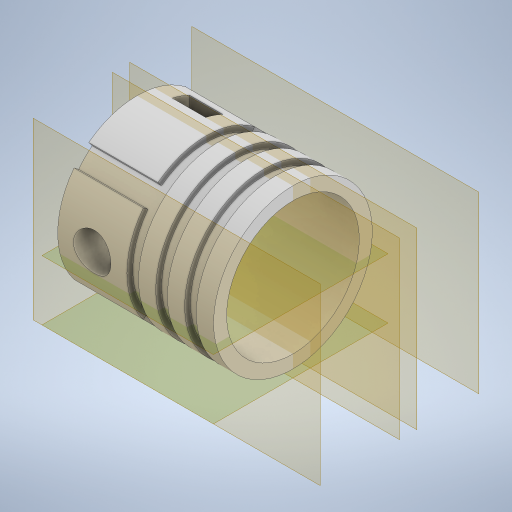
# Autodesk Inventor part: kolo_tetsowe
Saved by Autodesk Inventor 2023.5 (Build 275446000, 446)
## iProperties
Created: 2025-01-11
Part Number: kolo_tetsowe
Material: Ogólny
Document SubType Name: Modeling
Designer: kamil
Density: 1 g/cm^3
Appearance: Domyślna
Author: kamil
Autodesk Inventor part; units mm, degrees
ref_plane "YZ Plane" through (0, 0, 0) normal (1, 0, 0) x (0, 1, 0)
ref_plane "XZ Plane" through (0, 0, 0) normal (0, 1, 0) x (-1, 0, 0)
sketch "Szkic1" plane through (0, 0, 0) normal (1, 0, 0) x (0, 1, 0)
  circle A0 centre (0, 0) radius 16
  dimension "d0" = 32
  constraints: 1 centre point, 1 coincident
  measures "d0" diameter of A0
extrude "Wyciągnięcie proste1" add sketch "Szkic1" along normal blind 28
sketch "Szkic2" plane through (0, 0, 0) normal (-1, 0, 0) x (0, 0, 1)
  circle A0 centre (0, 0) radius 11.5
  dimension "d3" = 23
  constraints: 1 centre point, 1 coincident
  measures "d3" diameter of A0
extrude "Wyciągnięcie proste2" cut sketch "Szkic2" against normal blind 30.8
sketch "Szkic3" plane through (0, 0, 0) normal (-1, 0, 0) x (0, 0, 1)
  circle A0 centre (0, 0) radius 16 projected
extrude "Wyciągnięcie proste3" add sketch "Szkic3" against normal blind 2
sketch "Szkic4" plane through (0, 0, 0) normal (-1, 0, 0) x (0, 0, 1)
  circle A0 centre (0, 0) radius 1.8
  dimension "d8" = 3.6
  constraints: 1 centre point, 1 coincident
  measures "d8" diameter of A0
extrude "Wyciągnięcie proste4" cut sketch "Szkic4" against normal blind 28
sketch "Szkic5" plane through (2, 0, 0) normal (1, 0, 0) x (0, 0, -1)
  circle A0 centre (0, 0) radius 1.8 projected
  circle A1 centre (0, 0) radius 11.5 projected
extrude "Wyciągnięcie proste5" add sketch "Szkic5" along normal blind 9
sketch "Szkic6" plane through (28, 0, 0) normal (1, 0, 0) x (0, 0, -1)
  circle A0 centre (0, 0) radius 11.5 projected
  circle A1 centre (0, 0) radius 16 projected
  line L0 (-11.5, 0) -> (-16, 0)
  circle A2 centre (0, 0) radius 13.75
  point P0 (-13.75, 0)
  constraints: 4 horizontal alignment, 2 end point, 1 coincident, 1 horizontal, 1 midpoint, 4 other
extrude "Wyciągnięcie proste6" cut sketch "Szkic6" against normal through all contours A1
sketch "Szkic7" plane through (28, 0, 0) normal (1, 0, 0) x (0, 0, -1)
  circle A0 centre (0, 0) radius 13.75 projected
  circle A1 centre (0, 0) radius 11.5 projected
extrude "Wyciągnięcie proste7" add sketch "Szkic7" along normal blind 1
ref_plane "Płaszczyzna konstrukcyjna1" through (28, 0, 0) normal (0, 0, 1) x (1, 0, 0)
sketch "Szkic8" plane through (28, 0, 0) normal (0, 0, 1) x (1, 0, 0)
  line L0 (1, -13.75) -> (1, 13.75) projected
  line L1 (-28, 13.75) -> (-28, -13.75) projected
  line L2 (1, 11.5) -> (1, -11.5) projected
  line L3 (-17, 11.5) -> (-17, -11.5) projected
  line L4 (-19, 7.6749) -> (-19, -7.6749)
  line L5 (-28, 13.75) -> (1, 13.75) projected
  line L6 (-28, 13.75) -> (-19, 13.75)
  line L7 (-19, 13.75) -> (-19, 11.75)
  line L8 (-19, 11.75) -> (-28, 11.75)
  line L9 (-28, 11.75) -> (-28, 13.75)
  line L10 (-26, 11.75) -> (-26, 13.75)
  line L11 (-23.5, 13.75) -> (-23.5, 11.75)
  line L12 (-21.5, 13.75) -> (-21.5, 11.75)
  line L13 (-28, 0) -> (-19, 0)
  point P0 (-17, 0)
  point P1 (-19, 13.75)
  dimension "d17" = 2
  dimension "d18" = 2
  dimension "d19" = 2
  dimension "d20" = 2.5
  dimension "d21" = 2.5
  constraints: 18 end point, 5 point on line, 4 midpoint, 4 perpendicular, 3 parallel, 1 horizontal, 1 horizontal alignment
  measures "d17" distance between parallel lines of L3 L4
  measures "d18" distance of L6.end L7.end
  measures "d19" distance between parallel lines of L1 L10
  measures "d20" distance from line of L4.start L12
  measures "d21" distance between parallel lines of L10 L11
revolve "Obrót1" [suppressed]
sketch "Szkic9" plane through (11, 0, 0) normal (1, 0, 0) x (0, 0, -1)
  circle A0 centre (0, 0) radius 11.5 projected
  circle A1 centre (0, 0) radius 1.8 projected
extrude "Wyciągnięcie proste8" add sketch "Szkic9" along normal blind 0.5
sketch "Szkic10" plane through (28, 0, 0) normal (0, 0, 1) x (1, 0, 0)
  line L0 (-23.15, -1) -> (-23.15, 1) projected
  line L1 (-16.9, 1) -> (-16.9, -1) projected
  line L2 (-23.15, 0) -> (-16.9, 0)
  circle A0 centre (-20.025, 0) radius 1.4
  point P0 (-28, 0)
  dimension "d25" = 2.8
  constraints: 3 midpoint, 2 end point, 1 centre point
  measures "d25" diameter of A0
extrude "Wyciągnięcie proste9" cut sketch "Szkic10" along normal mid plane 30
ref_plane "Płaszczyzna konstrukcyjna2" through (28, 0, -13.75) normal (0, 0, 1) x (1, 0, 0)
sketch "Szkic11" plane through (28, 0, -13.75) normal (0, 0, 1) x (1, 0, 0)
  circle A0 centre (-20.025, 0) radius 1.4
  point P0 (-28, 0)
  constraints: 2 coincident, 1 centre point, 2 other
hole "Otwór1" at (7.975, 0, -13.75) direction (0, 0, 1) diameter 3.2 end through all counterbore diameter 6.5 counterbore depth 6
ref_plane "Płaszczyzna konstrukcyjna3" through (28, 0, -3) normal (0, 0, 1) x (1, 0, 0)
sketch "Szkic12" plane through (28, 0, -3) normal (0, 0, 1) x (1, 0, 0)
  circle A0 centre (-20.025, 0) radius 1.6 projected
  circle A1 centre (-20.025, 0) radius 2.9
  line L0 (-22.925, 1.6743) -> (-20.025, 3.3486)
  line L1 (-20.025, 3.3486) -> (-17.125, 1.6743)
  line L2 (-17.125, 1.6743) -> (-17.125, -1.6743)
  line L3 (-17.125, -1.6743) -> (-20.025, -3.3486)
  line L4 (-20.025, -3.3486) -> (-22.925, -1.6743)
  line L5 (-22.925, -1.6743) -> (-22.925, 1.6743)
  line L6 (-22.925, 17.3819) -> (-17.125, 17.3819)
  line L7 (-17.125, 17.3819) -> (-17.125, 1.6743)
  line L8 (-17.125, 1.6743) -> (-22.925, 1.6743)
  line L9 (-22.925, 1.6743) -> (-22.925, 17.3819)
  point P0 (-28, 0)
  point P1 (-22.925, 0)
  dimension "d36" = 5.8
  constraints: 20 end point, 2 coincident, 2 parallel, 1 horizontal, 1 horizontal alignment, 1 midpoint, 1 perpendicular, 15 other
extrude "Wyciągnięcie proste10" cut sketch "Szkic12" against normal blind 3 contours A0 | A1 L8 | L2 L3 A1 | A1 L8 L2 | L8 A1 | A1 L1 L8 | L3 L4 A1 | L1 L0 L9 L6 L7 | A1 L0 L1 | L8 L0 A1 | A1 L5 L8 | L4 L5 A1
sketch "Szkic13" plane through (28, 0, 0) normal (0, 0, 1) x (1, 0, 0)
  line L0 (-28, 13.75) -> (1, 13.75) projected
  line L1 (-16.5, 11.5) -> (-16.5, -11.5) projected
  line L2 (1, 11.5) -> (1, -11.5) projected
  line L3 (1, 0) -> (-16.5, 0)
  line L4 (-16.5, 1.8) -> (-16.5, -1.8) projected
  line L5 (-2, 13.75) -> (-4, 13.75)
  line L6 (-4, 13.75) -> (-4, 12.75)
  line L7 (-4, 12.75) -> (-2, 12.75)
  line L8 (-2, 12.75) -> (-2, 13.75)
  line L9 (-7, 13.75) -> (-9, 13.75)
  line L10 (-9, 13.75) -> (-9, 12.75)
  line L11 (-9, 12.75) -> (-7, 12.75)
  line L12 (-7, 12.75) -> (-7, 13.75)
  line L13 (-12, 13.75) -> (-14, 13.75)
  line L14 (-14, 13.75) -> (-14, 12.75)
  line L15 (-14, 12.75) -> (-12, 12.75)
  line L16 (-12, 12.75) -> (-12, 13.75)
  point P0 (-28, 0)
  point P1 (-2, 13.25)
  point P2 (-7, 13.25)
  point P3 (-12, 13.25)
  point P4 (-9, 13.25)
  point P5 (-14, 13.75)
  point P6 (-9, 13.75)
  point P7 (-4, 13.75)
  dimension "d39" = 2
  dimension "d40" = 1
  dimension "d41" = 2
  dimension "d42" = 1
  dimension "d43" = 2
  dimension "d44" = 1
  dimension "d45" = 3
  dimension "d46" = 3
  dimension "d47" = 3
  constraints: 26 end point, 6 midpoint, 6 parallel, 3 horizontal, 3 perpendicular, 3 point on line
  measures "d39" distance of L7.end L6.end
  measures "d40" distance of L6.end L5.end
  measures "d41" distance of L11.end L10.end
  measures "d42" distance of L10.end L9.end
  measures "d43" distance of L15.end L14.end
  measures "d44" distance of L14.end L13.end
  measures "d45" horizontal distance of point (-2, 13.25) L0.end
  measures "d46" distance from line of point (-7, 13.25) L6
  measures "d47" distance of point (-12, 13.25) point (-9, 13.25)
revolve "Obrót2" cut sketch "Szkic13" angle 360 about axis through (29, 0, 0) along (-1, 0, 0)
fillet "Zaokrąglenie1" radius 1 1 edges at (11.5, 0, -11.5)
ref_plane "Płaszczyzna konstrukcyjna4" through (28, 0, 13.75) normal (0, 0, 1) x (1, 0, 0)
sketch "Szkic14" plane through (28, 0, 13.75) normal (0, 0, 1) x (1, 0, 0)
  circle A0 centre (-20.025, 0) radius 1.4
  point P0 (-28, 0)
  dimension "d50" = 2.8
  constraints: 2 coincident, 1 centre point, 1 other
  measures "d50" diameter of A0
hole "Otwór2" at (7.975, 0, 13.75) direction (0, 0, -1) diameter 2.8 depth 14 tip angle 118 counterbore diameter 6.5 counterbore depth 5
sketch "Szkic15" plane through (0, 0, 0) normal (-1, 0, 0) x (0, 0, 1)
  circle A0 centre (0, 0) radius 13.75 projected
  circle A1 centre (0, 0) radius 1.8 projected
extrude "Wyciągnięcie proste11" cut sketch "Szkic15" against normal blind 2
ref_plane "Płaszczyzna konstrukcyjna8" through (28, -13.75, 0) normal (0, -1, 0) x (0, 0, -1)
ref_plane "Płaszczyzna konstrukcyjna7" through (7.975, -3.3486, -3) normal (0, -1, 0) x (0, 0, -1)
sketch "Szkic16" plane through (28, -13.75, 0) normal (0, -1, 0) x (0, 0, -1)
  line L0 (-8.75, -18.625) -> (-8.75, -21.425) projected
  line L1 (-1.8, -26) -> (1.8, -26) projected
  line L2 (-1.8, -16.5) -> (1.8, -16.5) projected
  line L3 (-1.8, -16.5) -> (1.8, -16.5) projected
  line L4 (-1.8, -26) -> (1.8, -26) projected
  line L5 (0, -26) -> (0, -16.5)
  line L6 (-8.75, -16.775) -> (-8.75, -23.275) projected
  line L7 (-8.75, -20.025) -> (0, -20.025)
  point P0 (0, -28)
  point P1 (-1.1314, -20.025)
  point P2 (0.8246, -20.025)
  constraints: 4 end point, 3 midpoint, 1 coincident, 1 perpendicular, 1 point on line
hole "Otwór3" at (7.975, -13.75, 0) direction (0, 1, 0) diameter 2.8 depth 14 tip angle 118 counterbore diameter 6.5 counterbore depth 5
sketch "Szkic17" plane through (2, 0, 0) normal (-1, 0, 0) x (0, 0, 1)
  circle A0 centre (0, 0) radius 13.75 projected
  circle A1 centre (0, 0) radius 12.75
  line L0 (0, 0) -> (10.9086, 8.3705)
  line L1 (0, 0) -> (8.3705, 10.9086)
  line L2 (0, 0) -> (12.75, 0)
  point P0 (7.7617, 10.1153)
  point P1 (10.1153, 7.7617)
  dimension "d68" = 1
  dimension "d69" = 15
  dimension "d70" = 37.5
  constraints: 6 end point, 2 point on circle, 1 horizontal, 3 other
  measures "d69" angle of L1 L0
  measures "d70" angle of L0 L2
extrude "Wyciągnięcie proste12" cut sketch "Szkic17" against normal up to surface (14 mm away) contours L0 A1 L1 A0 picked at (10.3871, 8.4739)
pattern_circular "Szyk kołowy1" count 4 over 360 about axis through (28, 0, 0) along (-1, 0, 0) of "Wyciągnięcie proste12"
sketch "Szkic18" plane through (2, 0, 0) normal (-1, 0, 0) x (0, 0, 1)
  circle A0 centre (0, 0) radius 1 projected
  circle A1 centre (0, 0) radius 1.8 projected
  circle A2 centre (0, 0) radius 1.2494
  constraints: 1 centre point
ref_plane "Płaszczyzna konstrukcyjna9" through (4.85, -1.8, -1.8) normal (-1, 0, 0) x (0, 0, 1)
extrude "Wyciągnięcie proste13" add sketch "Szkic18" against normal up to surface (2.85 mm away) contours A1
sketch "Szkic19" plane through (11.5, 0, 0) normal (1, 0, 0) x (0, 0, -1)
  circle A0 centre (0, 0) radius 1.8 projected
  circle A1 centre (0, 0) radius 1.9
  dimension "d78" = 0.1
  constraints: 1 centre point
  measures "d78" radial gap between concentric circles of A0 A1
extrude "Wyciągnięcie proste14" cut sketch "Szkic19" against normal up to surface (6.65 mm away) contours A0 | A1
chamfer "Faza1" distance 0.5 angle 45 1 edges at (11.5, 0, 1.9)
chamfer "Faza2" distance 0.5 angle 45 2 edges at (7.975, -1.6, -7.75) (7.975, -8.75, 1.4)
sketch "Szkic20" plane through (11.5, 0, 0) normal (1, 0, 0) x (0, 0, -1)
  circle A0 centre (0, 0) radius 2.4 projected
extrude "Wyciągnięcie proste15" add sketch "Szkic20" against normal up to surface (9.5 mm away)
sketch "Szkic21" plane through (2, 0, 0) normal (-1, 0, 0) x (0, 0, 1)
  circle A0 centre (0, 0) radius 1.5
  line L0 (-1, 1.118) -> (-1, -1.118)
  dimension "d89" = 3
  dimension "d90" = 1
  constraints: 2 end point, 2 point on circle, 1 centre point, 1 coincident, 1 vertical
  measures "d89" diameter of A0
  measures "d90" distance from line of L0 point (0, 0)
extrude "Wyciągnięcie proste16" cut sketch "Szkic21" against normal through all contours A0 L0 picked at (-0.1667, 0)
sketch "Szkic22" plane through (7.975, 0, -7.75) normal (0, 0, -1) x (-1, 0, 0)
  circle A0 centre (0, 0) radius 1.6 projected
  point P0 (7.975, 0)
extrude "Wyciągnięcie proste17" cut sketch "Szkic22" against normal through all
sketch "Szkic23" plane through (7.975, -8.75, 0) normal (0, -1, 0) x (1, 0, 0)
  circle A0 centre (0, 0) radius 1.4 projected
  point P0 (-7.975, 0)
extrude "Wyciągnięcie proste18" cut sketch "Szkic23" against normal blind 8
sketch "Szkic24" plane through (2, 0, 0) normal (-1, 0, 0) x (0, 0, 1)
  arc A0 (-1, -1.118) -> (-1, 1.118) centre (0, 0) ccw projected
  line L0 (-1, -1.118) -> (-1, 1.118) projected
  arc A1 (-1.2, -1.2042) -> (-1.2, 1.2042) centre (0, 0) ccw
  line L1 (-1.2, -1.2042) -> (-1.2, 1.2042)
  dimension "d97" = 0.2
  constraints: 2 end point, 2 point on circle, 1 centre point, 1 other
  measures "d97" radial gap between concentric circles of A0 A1
extrude "Wyciągnięcie proste19" cut sketch "Szkic24" against normal through all contours L0 A0 | L1 A1
sketch "Szkic25" plane through (11.5, 0, 0) normal (1, 0, 0) x (0, 0, -1)
  line L0 (7.9941, 15.6689) -> (7.9941, -15.6689) construction
  line L1 (7.9941, -15.6689) -> (1.4789, -15.6689) construction
  line L2 (1.4789, -15.6689) -> (1.4789, 15.6689) construction
  line L3 (1.4789, 15.6689) -> (7.9941, 15.6689) construction
  line L4 (1.2, 1.2042) -> (1.2, -1.2042) projected
  spline S0 degree 2 poles (4.7385, 3.5271) (4.0902, 3.5271) (3.1178, 3.7338) (2.7896, 3.9647) knots 0 0 0 1 2 2 2
  spline S1 degree 2 poles (2.7896, 3.9647) (2.4654, 4.1917) (2.1332, 4.925) (2.1332, 5.4518) knots 0 0 0 1 2 2 2
  spline S2 degree 2 poles (2.1332, 5.4518) (2.1332, 5.9826) (2.4654, 6.7119) (2.7977, 6.9429) knots 0 0 0 1 2 2 2
  spline S3 degree 2 poles (2.7977, 6.9429) (3.1259, 7.1738) (4.0902, 7.3805) (4.7385, 7.3805) knots 0 0 0 1 2 2 2
  spline S4 degree 2 poles (4.7385, 7.3805) (5.403, 7.3805) (6.343, 7.1738) (6.6834, 6.9388) knots 0 0 0 1 2 2 2
  spline S5 degree 2 poles (6.6834, 6.9388) (7.0157, 6.7038) (7.3398, 5.9623) (7.3398, 5.4518) knots 0 0 0 1 2 2 2
  spline S6 degree 2 poles (7.3398, 5.4518) (7.3398, 4.9129) (6.9994, 4.1917) (6.6631, 3.9607) knots 0 0 0 1 2 2 2
  spline S7 degree 2 poles (6.6631, 3.9607) (6.3349, 3.7338) (5.3665, 3.5271) (4.7385, 3.5271) knots 0 0 0 1 2 2 2
  spline S8 degree 2 poles (4.7385, 4.7873) (5.6664, 4.7873) (6.416, 5.0912) (6.416, 5.4518) knots 0 0 0 1 2 2 2
  spline S9 degree 2 poles (6.416, 5.4518) (6.416, 5.8124) (5.6664, 6.1203) (4.7345, 6.1203) knots 0 0 0 1 2 2 2
  spline S10 degree 2 poles (4.7345, 6.1203) (3.8187, 6.1203) (3.057, 5.8124) (3.057, 5.4518) knots 0 0 0 1 2 2 2
  spline S11 degree 2 poles (3.057, 5.4518) (3.057, 5.0952) (3.8187, 4.7873) (4.7385, 4.7873) knots 0 0 0 1 2 2 2
  line L5 (2.2385, 1.5985) -> (2.2385, 2.7857)
  line L6 (2.2385, 2.7857) -> (3.5594, 2.7857)
  line L7 (3.5594, 2.7857) -> (3.5594, 1.5985)
  line L8 (3.5594, 1.5985) -> (2.2385, 1.5985)
  line L9 (2.2385, -3.0652) -> (2.2385, 0.6098)
  line L10 (2.2385, 0.6098) -> (3.0529, 0.6098)
  spline S12 degree 2 poles (3.0529, 0.6098) (3.4257, 0.1438) (4.0821, -0.6017) (4.3779, -0.8813) knots 0 0 0 1 2 2 2
  spline S13 degree 2 poles (4.3779, -0.8813) (4.7628, -1.25) (5.3503, -1.5782) (5.6583, -1.5782) knots 0 0 0 1 2 2 2
  spline S14 degree 2 poles (5.6583, -1.5782) (6.0067, -1.5782) (6.3795, -1.1609) (6.3795, -0.7881) knots 0 0 0 1 2 2 2
  spline S15 degree 2 poles (6.3795, -0.7881) (6.3795, -0.5977) (6.2863, -0.2573) (6.2134, -0.0831) knots 0 0 0 1 2 2 2
  spline S16 degree 2 poles (6.2134, -0.0831) (6.1364, 0.0871) (5.9743, 0.3302) (5.9338, 0.391) knots 0 0 0 1 2 2 2
  line L11 (5.9338, 0.391) -> (5.9338, 0.4882)
  line L12 (5.9338, 0.4882) -> (7.0238, 0.4882)
  spline S17 degree 2 poles (7.0238, 0.4882) (7.1251, 0.2776) (7.3358, -0.622) (7.3358, -1.0393) knots 0 0 0 1 2 2 2
  spline S18 degree 2 poles (7.3358, -1.0393) (7.3358, -1.9307) (6.5416, -2.8464) (5.8244, -2.8464) knots 0 0 0 1 2 2 2
  spline S19 degree 2 poles (5.8244, -2.8464) (5.3828, -2.8464) (4.5319, -2.4291) (4.0456, -1.9469) knots 0 0 0 1 2 2 2
  spline S20 degree 2 poles (4.0456, -1.9469) (3.7458, -1.643) (3.2798, -1.0717) (3.1826, -0.9461) knots 0 0 0 1 2 2 2
  line L13 (3.1826, -0.9461) -> (3.1826, -3.0652)
  line L14 (3.1826, -3.0652) -> (2.2385, -3.0652)
  spline S21 degree 2 poles (4.7385, -7.3805) (4.0902, -7.3805) (3.1178, -7.1738) (2.7896, -6.9429) knots 0 0 0 1 2 2 2
  spline S22 degree 2 poles (2.7896, -6.9429) (2.4654, -6.716) (2.1332, -5.9826) (2.1332, -5.4558) knots 0 0 0 1 2 2 2
  spline S23 degree 2 poles (2.1332, -5.4558) (2.1332, -4.925) (2.4654, -4.1957) (2.7977, -3.9647) knots 0 0 0 1 2 2 2
  spline S24 degree 2 poles (2.7977, -3.9647) (3.1259, -3.7338) (4.0902, -3.5271) (4.7385, -3.5271) knots 0 0 0 1 2 2 2
  spline S25 degree 2 poles (4.7385, -3.5271) (5.403, -3.5271) (6.343, -3.7338) (6.6834, -3.9688) knots 0 0 0 1 2 2 2
  spline S26 degree 2 poles (6.6834, -3.9688) (7.0157, -4.2038) (7.3398, -4.9453) (7.3398, -5.4558) knots 0 0 0 1 2 2 2
  spline S27 degree 2 poles (7.3398, -5.4558) (7.3398, -5.9947) (6.9994, -6.716) (6.6631, -6.9469) knots 0 0 0 1 2 2 2
  spline S28 degree 2 poles (6.6631, -6.9469) (6.3349, -7.1738) (5.3665, -7.3805) (4.7385, -7.3805) knots 0 0 0 1 2 2 2
  spline S29 degree 2 poles (4.7385, -6.1203) (5.6664, -6.1203) (6.416, -5.8165) (6.416, -5.4558) knots 0 0 0 1 2 2 2
  spline S30 degree 2 poles (6.416, -5.4558) (6.416, -5.0952) (5.6664, -4.7873) (4.7345, -4.7873) knots 0 0 0 1 2 2 2
  spline S31 degree 2 poles (4.7345, -4.7873) (3.8187, -4.7873) (3.057, -5.0952) (3.057, -5.4558) knots 0 0 0 1 2 2 2
  spline S32 degree 2 poles (3.057, -5.4558) (3.057, -5.8124) (3.8187, -6.1203) (4.7385, -6.1203) knots 0 0 0 1 2 2 2
  point P0 (0, 0)
  point P1 (1.2, 0)
  point P2 (7.9941, 0)
  dimension "d97" = 0.2
  constraints: 2 midpoint, 1 horizontal alignment, 2 other
extrude "Wyciągnięcie proste20" cut sketch "Szkic25" against normal blind 0.5
chamfer "Faza3" distance 0.5 angle 45 2 edges at (11.5, 0, 1.7) (11.5, 0, -1.2)
